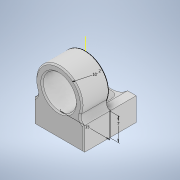
# Autodesk Inventor part: cable_managerr
Saved by Autodesk Inventor 2021 (Build 250183000, 183)
## iProperties
Created: 2020-09-06
Part Number: cable_managerr
Material: Generic
Document SubType Name: Modeling
Designer: Johansson
Density: 1 g/cm^3
Appearance: Default
Author: Johansson
## iProperties of the stored document _3DPrint.ipt
Created: 2020-09-06
Part Number: _3DPrint
Material: Generic
Document SubType Name: Modeling
Designer: Johansson
Density: 1 g/cm^3
Appearance: Default
Author: Johansson
Autodesk Inventor part; units mm, degrees
ref_plane "YZ Plane" through (0, 0, 0) normal (1, 0, 0) x (0, 1, 0)
ref_plane "XZ Plane" through (0, 0, 0) normal (0, 1, 0) x (-1, 0, 0)
ref_plane "XY Plane" through (0, 0, 0) normal (0, 0, 1) x (1, 0, 0)
sketch "Sketch1" plane through (0, 0, 0) normal (0, 0, 1) x (1, 0, 0)
  circle A0 centre (0, 8.5) radius 5
  circle A1 centre (0, 8.5) radius 7
  line L0 (-7.5, -3.5) -> (7.5, -3.5)
  line L1 (7.5, -3.5) -> (7.5, 3.5)
  line L2 (7.5, 3.5) -> (-7.5, 3.5)
  line L3 (-7.5, 3.5) -> (-7.5, -3.5)
  line L4 (-7.5, -3.5) -> (7.5, 3.5) construction
  line L5 (7.5, -3.5) -> (-7.5, 3.5) construction
  line L6 (0, -7.3) -> (0, 19.3) projected
  point P0 (0, 0)
  point P1 (-4.899, 3.5)
  point P2 (4.899, 3.5)
  dimension "d0" = 10
  dimension "d1" = 2
  dimension "d2" = 7
  dimension "d3" = 15
  constraints: 12 end point, 2 centre point, 2 midpoint, 2 parallel, 1 coincident, 1 horizontal, 1 perpendicular, 1 point on line, 1 tangent
  measures "d0" diameter of A0
  measures "d1" radial gap between concentric circles of A0 A1
  measures "d2" distance of L0.end L1.end
  measures "d3" distance of L0.start L0.end
extrude "Extrusion1" add sketch "Sketch1" along normal blind 8 contours A0 L6 A1 L2 | A0 L2 A1 L6 | L6 A1 L2 | L2 A1 L6 | L2 L1 L0 L6 A1 | A1 L6 L0 L3 L2
extrude "Extrusion2" add sketch "Sketch1" against normal blind 8 contours L2 L1 L0 L6 A1 | A1 L6 L0 L3 L2
sketch "Sketch2" plane through (-7.5, -3.5, 8) normal (0, -1, 0) x (1, 0, 0)
  circle A0 centre (7.5, -12) radius 1.6
  point P0 (7.5, -8)
  dimension "d8" = 3.2
  constraints: 1 centre point, 1 coincident
  measures "d8" diameter of A0
extrude "Extrusion3" cut sketch "Sketch2" against normal up to next
chamfer "Chamfer1" distance 2 angle 45 1 edges at (-1.6, 1.6853, -3.9955)
fillet "Fillet1" radius 2 2 edges at (-4.899, 3.5, 4) (4.899, 3.5, 4)
fillet "Fillet2" radius 0.4 3 edges at (0, 1.5, 0) (-6.1995, 3.5, 0) (6.1995, 3.5, 0)
chamfer "Chamfer2" distance 0.4 angle 45 7 edges at (6.5392, 4.5643, 8) (0, 15.5, 8) (-6.5392, 4.5643, 8) (7.5, 0, 8) (0, -3.5, 8) (-7.5, 0, 8) (-5, 8.5, 8)
body "Solid1"
